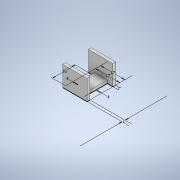
# Autodesk Inventor part: drzakCudliku
Saved by Autodesk Inventor 2022 (Build 260153000, 153)
## iProperties
Created: 2022-06-11
Part Number: drzakCudliku
Material: Generic
Document SubType Name: Modeling
Designer: adam
Density: 1 g/cm^3
Appearance: Default
Author: adam
Autodesk Inventor part; units mm, degrees
ref_plane "YZ Plane" through (0, 0, 0) normal (1, 0, 0) x (0, 1, 0)
ref_plane "XZ Plane" through (0, 0, 0) normal (0, 1, 0) x (-1, 0, 0)
ref_plane "XY Plane" through (0, 0, 0) normal (0, 0, 1) x (1, 0, 0)
sketch "Sketch1" plane through (0, 0, 0) normal (0, 1, 0) x (-1, 0, 0)
  line L0 (0, 0) -> (-17, 0)
  line L1 (-17, 0) -> (-17, -2)
  line L2 (-17, -2) -> (0, -2)
  line L3 (0, -2) -> (0, 0)
  line L4 (0, -18) -> (-17, -18)
  line L5 (-17, -18) -> (-17, -20)
  line L6 (-17, -20) -> (0, -20)
  line L7 (0, -20) -> (0, -18)
  line L8 (-4, -2) -> (-13, -2)
  line L9 (-13, -2) -> (-13, -18)
  line L10 (-13, -18) -> (-4, -18)
  line L11 (-4, -18) -> (-4, -2)
  dimension "d0" = 17
  dimension "d1" = 2
  dimension "d2" = 17
  dimension "d3" = 2
  dimension "d4" = 16
  dimension "d7" = 4
  dimension "d8" = 4
  constraints: 24 end point, 6 parallel, 3 horizontal, 3 perpendicular, 2 point on line
  measures "d0" distance of L2.end L1.end
  measures "d1" distance of L1.end L0.end
  measures "d2" distance of L6.end L5.end
  measures "d3" distance of L5.end L4.end
  measures "d4" distance between parallel lines of L4 L2
  measures "d7" distance from line of L2.end L11
  measures "d8" distance of L1.end L8.end
extrude "Extrusion1" add sketch "Sketch1" along normal blind 14 contours L3 L2 L1 L0 | L4 L7 L6 L5
extrude "Extrusion2" add sketch "Sketch1" along normal blind 2 contours L11 L4 L9 L2
body "Solid1"
